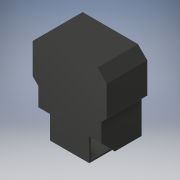
# Autodesk Inventor part: XT-LG-05
Saved by Autodesk Inventor 2017 SP1 (Build 210196100, 196)
## iProperties
Created: 2019-11-11
Part Number: XT-LG-05
Material: ABS Plastic
Document SubType Name: Modeling
Designer: Zach
Density: 1.06 g/cm^3
Appearance: Smooth - Black
Author: Zach
Autodesk Inventor part; units mm, degrees
ref_plane "YZ Plane" through (0, 0, 0) normal (1, 0, 0) x (0, 1, 0)
ref_plane "XZ Plane" through (0, 0, 0) normal (0, 1, 0) x (-1, 0, 0)
ref_plane "XY Plane" through (0, 0, 0) normal (0, 0, 1) x (1, 0, 0)
sketch "Sketch1" plane through (0, 0, 0) normal (0, 0, 1) x (1, 0, 0)
  line L0 (-60.1273, 59) -> (60.1273, 59)
  line L1 (-60.1273, 59) -> (-80.1273, 39)
  line L2 (-80.1273, 39) -> (-80.1273, -28)
  line L3 (-68.1273, -40) -> (-80.1273, -28)
  line L4 (-68.1273, -110) -> (-68.1273, -40)
  line L5 (-68.1273, -110) -> (-48.1273, -130)
  line L6 (-48.1273, -130) -> (48.1273, -130)
  line L7 (48.1273, -130) -> (68.1273, -110)
  line L8 (68.1273, -40) -> (68.1273, -110)
  line L9 (80.1273, -28) -> (68.1273, -40)
  line L10 (80.1273, 39) -> (80.1273, -28)
  line L11 (60.1273, 59) -> (80.1273, 39)
  point P0 (0, 0)
  point P1 (0, 0)
  constraints: 24 end point
extrude "Extrusion1" add sketch "Sketch1" along normal blind 3
sketch "Sketch2" plane through (0, 0, 0) normal (0, 0, -1) x (-1, 0, 0)
  line L0 (60.1273, 59) -> (-60.1273, 59) projected
  line L1 (-60.1273, 59) -> (-80.1273, 39) projected
  line L2 (-80.1273, 39) -> (-80.1273, -28) projected
  line L3 (-80.1273, -28) -> (-68.1273, -40) projected
  line L4 (-68.1273, -40) -> (-68.1273, -110) projected
  line L5 (-68.1273, -110) -> (-48.1273, -130) projected
  line L6 (-48.1273, -130) -> (48.1273, -130) projected
  line L7 (48.1273, -130) -> (68.1273, -110) projected
  line L8 (68.1273, -110) -> (68.1273, -40) projected
  line L9 (68.1273, -40) -> (80.1273, -28) projected
  line L10 (80.1273, -28) -> (80.1273, 39) projected
  line L11 (80.1273, 39) -> (60.1273, 59) projected
  line L12 (-59.2575, 56.9) -> (59.2575, 56.9)
  line L13 (59.2575, 56.9) -> (78.0273, 38.1302)
  line L14 (78.0273, 38.1302) -> (78.0273, -27.1302)
  line L15 (78.0273, -27.1302) -> (66.0273, -39.1302)
  line L16 (66.0273, -39.1302) -> (66.0273, -109.1302)
  line L17 (66.0273, -109.1302) -> (47.2575, -127.9)
  line L18 (47.2575, -127.9) -> (-47.2575, -127.9)
  line L19 (-47.2575, -127.9) -> (-66.0273, -109.1302)
  line L20 (-66.0273, -109.1302) -> (-66.0273, -39.1302)
  line L21 (-66.0273, -39.1302) -> (-78.0273, -27.1302)
  line L22 (-78.0273, -27.1302) -> (-78.0273, 38.1302)
  line L23 (-78.0273, 38.1302) -> (-59.2575, 56.9)
  point P0 (0, 0)
  dimension "d2" = 2.1
  constraints: 24 end point, 11 other
  measures "d2" distance between parallel lines of L0 L12
extrude "Extrusion2" add sketch "Sketch2" along normal blind 85
chamfer "Chamfer1" distance 50 angle 45 1 edges at (0, -130, 3)
sketch "Sketch3" plane through (-68.1273, -80, 3) normal (0, -0.7071068, 0.7071068) x (1, 0, 0)
  line L0 (2.1, -41.1963) -> (2.1, -4.2426) projected
  line L1 (2.1, -4.2426) -> (134.1547, -4.2426) construction
  line L2 (134.1547, -4.2426) -> (134.1547, -41.1963) projected
  line L3 (134.1547, -41.1963) -> (115.3848, -67.7408) projected
  line L4 (115.3848, -67.7408) -> (20.8698, -67.7408) construction
  line L5 (20.8698, -67.7408) -> (2.1, -41.1963) projected
  line L6 (136.2547, -42.4264) -> (136.2547, 0) projected
  line L7 (136.2547, 0) -> (0, 0) projected
  line L8 (0, 0) -> (0, -42.4264) projected
  line L9 (0, -42.4264) -> (20, -70.7107) projected
  line L10 (20, -70.7107) -> (116.2547, -70.7107) projected
  line L11 (116.2547, -70.7107) -> (136.2547, -42.4264) projected
  line L12 (136.2547, 0) -> (0, 0) projected
  line L13 (20, -70.7107) -> (116.2547, -70.7107) projected
  line L14 (25.6273, 0) -> (110.6273, 0)
  line L15 (110.6273, 0) -> (110.6273, -70.7107)
  line L16 (110.6273, -70.7107) -> (25.6273, -70.7107)
  line L17 (25.6273, -70.7107) -> (25.6273, 0)
  line L18 (20, -70.7107) -> (25.6273, -70.7107)
  line L19 (25.6273, -70.7107) -> (25.6273, -67.7408)
  line L20 (115.3848, -67.7408) -> (20.8698, -67.7408) projected
  line L21 (20.8698, -67.7408) -> (25.6273, -67.7408)
  line L22 (25.6273, 0) -> (0, 0)
  line L23 (2.1, -4.2426) -> (134.1547, -4.2426) projected
  line L24 (2.1, -4.2426) -> (25.6273, -4.2426)
  line L25 (25.6273, -4.2426) -> (25.6273, 0)
  line L26 (110.6273, 0) -> (136.2547, 0)
  line L27 (110.6273, -4.2426) -> (134.1547, -4.2426)
  line L28 (134.1547, 26.778) -> (134.1547, -33.326) projected
  line L29 (110.6273, -4.2426) -> (110.6273, 0)
  line L30 (110.6273, -70.7107) -> (116.2547, -70.7107)
  line L31 (115.3848, -67.7408) -> (110.6273, -67.7408)
  line L32 (110.6273, -67.7408) -> (110.6273, -70.7107)
  point P0 (68.1273, 54.4472)
  point P1 (68.1273, 0)
  dimension "d8" = 85
  constraints: 32 end point, 10 point on line, 4 collinear, 4 perpendicular, 2 midpoint, 2 parallel, 2 vertical, 1 horizontal
  measures "d8" distance between parallel lines of L15 L17
extrude "Extrusion3" add sketch "Sketch3" against normal blind 3 contours L5 L20 L17 L10 L9 L8 L7 L23 L0 | L0 L23 L17 L20 L5 | L17 L7 L15 L23 | L23 L2 L3 L20 L15 | L15 L7 L28 L23 | L20 L3 L2 L28 L7 L6 L11 L10 L15
sketch "Sketch5" plane through (0, 0, 3) normal (0, 0, 1) x (1, 0, 0)
  line L0 (66.0273, -78.7574) -> (-66.0273, -78.7574) projected
  line L1 (48.1273, -130) -> (-48.1273, -130) projected
  line L2 (-42.5, -78.7574) -> (42.5, -78.7574)
  line L3 (42.5, -78.7574) -> (42.5, -130)
  line L4 (42.5, -130) -> (-42.5, -130)
  line L5 (-42.5, -130) -> (-42.5, -78.7574)
  point P0 (0, 0)
  point P1 (42.5, -83)
  point P2 (-42.5, -83)
  constraints: 8 end point, 4 point on line, 2 parallel, 1 horizontal, 1 perpendicular
extrude "Extrusion4" add sketch "Sketch5" against normal blind 3
sketch "Sketch7" plane through (-48.1273, -130, -85) normal (0, -1, 0) x (1, 0, 0)
  line L0 (90.6273, 88) -> (5.6273, 88) projected
  line L1 (5.6273, 88) -> (90.6273, 88)
  line L2 (90.6273, 88) -> (90.6273, 38)
  line L3 (90.6273, 38) -> (5.6273, 38)
  line L4 (5.6273, 38) -> (5.6273, 88)
  line L5 (0, 38) -> (96.2547, 38) projected
  point P0 (48.1273, 85)
  constraints: 8 end point, 2 parallel, 1 horizontal, 1 perpendicular, 1 point on line
extrude "Extrusion5" add sketch "Sketch7" against normal blind 3
body "Solid1"
